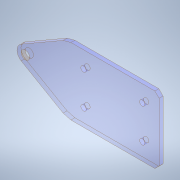
# Autodesk Inventor part: Papa John Mounting Plate
Saved by Autodesk Inventor 2020 (Build 240168000, 168)
## iProperties
Created: 2020-01-31
Part Number: Papa John Mounting Plate
Material: Polycarbonate, Smoke
Document SubType Name: Modeling
Designer: aidan
Density: 1.2 g/cm^3
Appearance: Polycarbonate - Smoked
Author: aidan
Autodesk Inventor part; units mm, degrees
ref_plane "YZ Plane" through (0, 0, 0) normal (1, 0, 0) x (0, 1, 0)
ref_plane "XZ Plane" through (0, 0, 0) normal (0, 1, 0) x (-1, 0, 0)
ref_plane "XY Plane" through (0, 0, 0) normal (0, 0, 1) x (1, 0, 0)
sketch "Sketch1" plane through (0, 0, 0) normal (0, 0, 1) x (1, 0, 0)
  line L0 (0, 0) -> (44.45, 0) construction
  line L1 (44.45, 0) -> (44.45, -25.4) construction
  line L2 (44.45, -25.4) -> (0, -25.4) construction
  line L3 (0, -25.4) -> (0, 0) construction
  line L4 (-12.7, 12.7) -> (57.15, 12.7)
  line L5 (57.15, 12.7) -> (57.15, -38.1)
  line L6 (57.15, -38.1) -> (-12.7, -38.1)
  line L7 (-12.7, 12.7) -> (-56.6941, -12.7)
  line L8 (-56.6941, -12.7) -> (-12.7, -38.1)
  dimension "d0" = 44.45
  dimension "d1" = 25.4
  dimension "d2" = 12.7
  dimension "d3" = 12.7
  dimension "d5" = 12.7
  constraints: 18 end point, 3 parallel, 2 horizontal, 2 perpendicular, 1 coincident, 1 equal length
  measures "d0" distance of L0.start L0.end
  measures "d1" distance of L0.end L1.end
  measures "d2" distance between parallel lines of L4 L0
  measures "d3" distance between parallel lines of L6 L2
  measures "d5" distance between parallel lines of L5 L1
extrude "Extrusion1" add sketch "Sketch1" along normal blind 2.9972
sketch "Sketch2" plane through (0, 0, 2.9972) normal (0, 0, 1) x (1, 0, 0)
  line L0 (0, -25.4) -> (44.45, -25.4) construction
  line L1 (44.45, -25.4) -> (44.45, 0) construction
  line L2 (44.45, 0) -> (0, 0) construction
  line L3 (0, 0) -> (0, -25.4) construction
  line L4 (-12.7, -38.1) -> (57.15, -38.1) projected
  line L5 (57.15, -38.1) -> (57.15, 12.7) projected
  circle A0 centre (0, 0) radius 2.0193
  circle A1 centre (44.45, 0) radius 2.0193
  circle A2 centre (44.45, -25.4) radius 2.0193
  circle A3 centre (0, -25.4) radius 2.0193
  point P0 (0, 0)
  dimension "d8" = 12.7
  dimension "d9" = 25.4
  dimension "d10" = 12.7
  dimension "d11" = 44.45
  dimension "d12" = 4.0386
  constraints: 8 end point, 4 centre point, 4 coincident, 3 equal radius, 2 parallel, 1 horizontal, 1 perpendicular
  measures "d8" distance between parallel lines of L4 L0
  measures "d9" distance of L0.end L1.end
  measures "d10" distance between parallel lines of L5 L1
  measures "d11" distance of L1.end L2.end
  measures "d12" diameter of A0
extrude "Extrusion2" cut sketch "Sketch2" against normal through all
fillet "Fillet1" radius 6.35 1 edges at (-56.6941, -12.7, 1.4986)
chamfer "Chamfer1" distance 3.175 angle 45 4 edges at (57.15, 12.7, 1.4986) (57.15, -38.1, 1.4986) (-12.7, 12.7, 1.4986) (-12.7, -38.1, 1.4986)
sketch "Sketch3" plane through (0, 0, 2.9972) normal (0, 0, 1) x (1, 0, 0)
  arc A0 (-47.1691, -7.2007) -> (-47.1691, -18.1993) centre (-43.9941, -12.7) ccw projected
  circle A1 centre (-43.9941, -12.7) radius 3.175
  point P0 (0, 0)
  dimension "d19" = 6.35
  constraints: 1 centre point, 1 coincident
  measures "d19" diameter of A1
hole "Hole1" at (-43.9941, -12.7, 2.9972) direction (0, 0, -1) diameter 6.35 end through all
body "Solid1"
